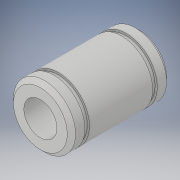
# Autodesk Inventor part: Linear Bearing 8mm
Saved by Autodesk Inventor 2019 (Build 230136000, 136)
## iProperties
Created: 2019-04-25
Part Number: Linear Bearing 8mm
Material: Generic
Document SubType Name: Modeling
Designer: 19879326
Density: 1 g/cm^3
Appearance: Default
Author: 19879326
Autodesk Inventor part; units mm, degrees
ref_plane "YZ Plane" through (0, 0, 0) normal (1, 0, 0) x (0, 1, 0)
ref_plane "XZ Plane" through (0, 0, 0) normal (0, 1, 0) x (-1, 0, 0)
ref_plane "XY Plane" through (0, 0, 0) normal (0, 0, 1) x (1, 0, 0)
sketch "Sketch1" plane through (0, 0, 0) normal (1, 0, 0) x (0, 1, 0)
  line L0 (4, 12) -> (4, -12)
  line L1 (4, -12) -> (7.5, -12)
  line L2 (7.5, -12) -> (7.5, -8.75)
  line L3 (7.5, -8.75) -> (7, -8.75)
  line L4 (7, -8.75) -> (7, -7.65)
  line L5 (7, -7.65) -> (7.5, -7.65)
  line L6 (7.5, -7.65) -> (7.5, 7.65)
  line L7 (7.5, 7.65) -> (7, 7.65)
  line L8 (7, 7.65) -> (7, 8.75)
  line L9 (7, 8.75) -> (7.5, 8.75)
  line L10 (7.5, 8.75) -> (7.5, 12)
  line L11 (7.5, 12) -> (4, 12)
  line L12 (0, -16.8) -> (0, 16.8) projected
  point P0 (0, 0)
  point P1 (4, 0)
  point P2 (7, -8.2)
  point P3 (7, 8.2)
  dimension "d0" = 1.1
  dimension "d1" = 1.1
  dimension "d2" = 15.3
  dimension "d3" = 3.25
  dimension "d4" = 3.25
  dimension "d5" = 4
  dimension "d6" = 7.5
  dimension "d7" = 7
  constraints: 24 end point, 9 perpendicular, 4 point on line, 3 midpoint, 1 horizontal alignment, 1 vertical, 1 vertical alignment
  measures "d0" distance of L7.end L8.end
  measures "d1" distance of L3.end L4.end
  measures "d2" distance of L5.end L6.end
  measures "d3" distance of L9.end L10.end
  measures "d4" distance of L1.end L2.end
  measures "d5" distance from line of L0 point (0, 0)
  measures "d6" distance from line of point (0, 0) L6
  measures "d7" distance from line of point (0, 0) L4
revolve "Revolution1" add sketch "Sketch1" angle 360 about axis through (0, 0, -10) along (0, 0, 1)
chamfer "Chamfer1" distance 1 angle 45 2 edges at (0, -7.5, 12) (0, -7.5, -12)
body "Solid1"
